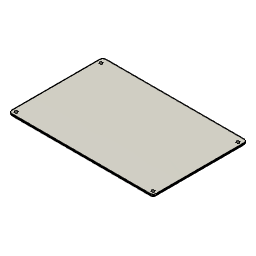
Simple Case V2 - Lid (Autodesk Fusion 360 design; units mm, degrees)
Autodesk Fusion 360 part; units mm, degrees
sketch "Sketch1" plane through (0, 0, 63) normal (0, 0, 1) x (-1, 0, 0)
  line L0 (-110, -73.4) -> (-107, -73.4)
  line L1 (-107, -73.4) -> (-107, -72)
  line L2 (-107, -72) -> (-99, -72)
  line L3 (-99, -72) -> (-99, -69)
  line L4 (-99, -69) -> (-103, -69)
  arc A0 (-106, -66) -> (-103, -69) centre (-103, -66) ccw
  arc A1 (-106, -66) -> (-109, -63) centre (-109, -66) ccw
  arc A2 (-112, -60) -> (-109, -63) centre (-109, -60) ccw
  line L5 (-112, -60) -> (-112, 63)
  arc A3 (-109, 66) -> (-112, 63) centre (-109, 63) ccw
  arc A4 (-109, 66) -> (-106, 69) centre (-109, 69) ccw
  arc A5 (-103, 72) -> (-106, 69) centre (-103, 69) ccw
  line L6 (-103, 72) -> (103, 72)
  arc A6 (106, 69) -> (103, 72) centre (103, 69) ccw
  arc A7 (106, 69) -> (109, 66) centre (109, 69) ccw
  arc A8 (112, 63) -> (109, 66) centre (109, 63) ccw
  line L7 (112, 63) -> (112, -60)
  arc A9 (109, -63) -> (112, -60) centre (109, -60) ccw
  arc A10 (109, -63) -> (106, -66) centre (109, -66) ccw
  arc A11 (103, -69) -> (106, -66) centre (103, -66) ccw
  line L8 (103, -69) -> (99, -69)
  line L9 (99, -69) -> (99, -72)
  line L10 (99, -72) -> (107, -72)
  line L11 (107, -72) -> (107, -73.4)
  line L12 (107, -73.4) -> (110, -73.4)
  arc A12 (110, -73.4) -> (113.4, -70) centre (110, -70) ccw
  line L13 (113.4, -70) -> (113.4, 70)
  arc A13 (113.4, 70) -> (110, 73.4) centre (110, 70) ccw
  line L14 (110, 73.4) -> (-110, 73.4)
  arc A14 (-110, 73.4) -> (-113.4, 70) centre (-110, 70) ccw
  line L15 (-113.4, 70) -> (-113.4, -70)
  arc A15 (-113.4, -70) -> (-110, -73.4) centre (-110, -70) ccw
  circle A16 centre (-109, -66) radius 1.925
  circle A17 centre (109, -66) radius 1.925
  circle A18 centre (109, 69) radius 1.925
  circle A19 centre (-109, 69) radius 1.925
  line L16 (107, -73.4) -> (-107, -73.4)
  line L17 (-99, -72) -> (99, -72)
  circle A20 centre (109, -66) radius 2.25
  circle A21 centre (109, 69) radius 2.25
  circle A22 centre (-109, 69) radius 2.25
  circle A23 centre (-109, -66) radius 2.25
  line L18 (107, -73.15) -> (-107, -73.15)
  line L19 (-110, -73.15) -> (-107, -73.15)
  arc A24 (-113.15, -70) -> (-110, -73.15) centre (-110, -70) ccw
  line L20 (-113.15, 70) -> (-113.15, -70)
  arc A25 (-110, 73.15) -> (-113.15, 70) centre (-110, 70) ccw
  line L21 (110, 73.15) -> (-110, 73.15)
  arc A26 (113.15, 70) -> (110, 73.15) centre (110, 70) ccw
  line L22 (113.15, -70) -> (113.15, 70)
  arc A27 (110, -73.15) -> (113.15, -70) centre (110, -70) ccw
  line L23 (107, -73.15) -> (110, -73.15)
  dimension "d149" = 4.5
  dimension "d150" = 4.5
  dimension "d151" = 4.5
  dimension "d152" = 4.5
  dimension "d153" = 0.25
  constraint coincident L11.end L12.start
  constraint coincident L0.end L1.start
  constraint coincident L2.end L3.start
  constraint coincident L9.end L10.start
  constraint concentric A10 A20
  constraint concentric A7 A21
  constraint concentric A4 A22
  constraint concentric A1 A23
  measures "d149" diameter of A20
  measures "d150" diameter of A21
  measures "d151" diameter of A22
  measures "d152" diameter of A23
extrude "Extrude1" add sketch "Sketch1" along normal blind 2.2 contours L1 L2 L3 L4 A0 A1 A2 L5 A3 A4 A5 L6 A6 A7 A8 L7 A9 A10 A11 L8 L9 L10 L11 L19 A24 L20 A25 L21 A26 L22 A27 L23 | L1 L2 L10 L11 L17 L18 | L3 L4 A0 A1 A2 L5 A3 A4 A5 L6 A6 A7 A8 L7 A9 A10 A11 L8 L9 L17
sketch "Sketch2" plane through (0, 0, 65.2) normal (0, 0, 1) x (-1, 0, 0)
  circle A0 centre (-109, 69) radius 2.25
  circle A1 centre (109, -66) radius 2.25
  circle A2 centre (109, 69) radius 2.25
  circle A3 centre (-109, -66) radius 2.25
  line L0 (-110, -73.15) -> (110, -73.15)
  arc A4 (110, -73.15) -> (113.15, -70) centre (110, -70) ccw
  line L1 (113.15, -70) -> (113.15, 70)
  arc A5 (113.15, 70) -> (110, 73.15) centre (110, 70) ccw
  line L2 (110, 73.15) -> (-110, 73.15)
  arc A6 (-110, 73.15) -> (-113.15, 70) centre (-110, 70) ccw
  line L3 (-113.15, 70) -> (-113.15, -70)
  arc A7 (-113.15, -70) -> (-110, -73.15) centre (-110, -70) ccw
  line L4 (-115, 70) -> (-115, -70)
  arc A8 (-115, -70) -> (-110, -75) centre (-110, -70) ccw
  line L5 (-107, -75) -> (107, -75)
  line L6 (-110, -75) -> (-107, -75)
  line L7 (107, -75) -> (110, -75)
  arc A9 (110, -75) -> (115, -70) centre (110, -70) ccw
  line L8 (115, -70) -> (115, 70)
  arc A10 (115, 70) -> (110, 75) centre (110, 70) ccw
  line L9 (110, 75) -> (-110, 75)
  arc A11 (-110, 75) -> (-115, 70) centre (-110, 70) ccw
extrude "Extrude2" add sketch "Sketch2" along normal blind 2 contours L0 A4 L1 A5 L2 A6 L3 A7 | L4 A8 L5 L6 L7 A9 L8 A10 L9 A11
move_body "Move1" bodies 1 to x (1, 0, 0) y (0, 1, 0) z (0, 0, 1) at (0, 0, 50)
